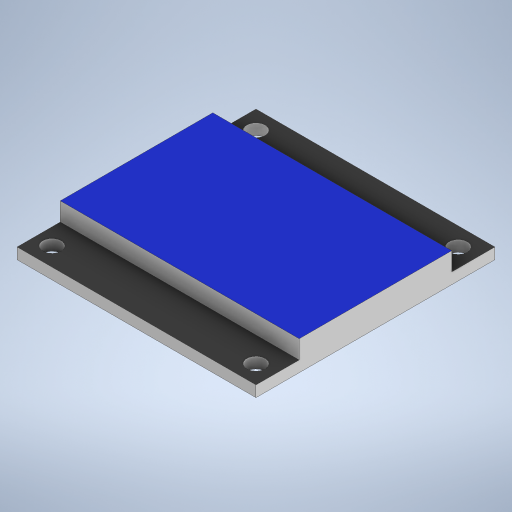
# Autodesk Inventor part: ssd1360
Saved by Autodesk Inventor 2023 (Build 270158000, 158)
## iProperties
Created: 2023-05-18
Part Number: ssd1360
Material: Generic
Document SubType Name: Modeling
Designer: mark
Density: 1 g/cm^3
Appearance: Default
Author: mark
Autodesk Inventor part; units mm, degrees
ref_plane "YZ Plane" through (0, 0, 0) normal (1, 0, 0) x (0, 1, 0)
ref_plane "XZ Plane" through (0, 0, 0) normal (0, 1, 0) x (-1, 0, 0)
ref_plane "XY Plane" through (0, 0, 0) normal (0, 0, 1) x (1, 0, 0)
sketch "Sketch1" plane through (0, 0, 0) normal (0, 1, 0) x (-1, 0, 0)
  line L0 (63.6448, -68.929) -> (37.6448, -68.929)
  line L1 (37.6448, -68.929) -> (37.6448, -42.929)
  line L2 (37.6448, -42.929) -> (63.6448, -42.929)
  line L3 (63.6448, -42.929) -> (63.6448, -68.929)
  point P0 (0, 0)
  dimension "d0" = 26
  dimension "d1" = 26
  constraints: 8 end point, 2 parallel, 1 horizontal, 1 perpendicular
  measures "d0" distance of L1.end L2.end
  measures "d1" distance of L0.end L1.end
extrude "Extrusion1" add sketch "Sketch1" along normal blind 1.2
sketch "Sketch2" plane through (0, 1.2, 0) normal (0, 1, 0) x (1, 0, 0)
  line L0 (-63.6448, 68.929) -> (-63.6448, 42.929) projected
  line L1 (-37.6448, 42.929) -> (-37.6448, 68.929) projected
  line L2 (-63.6448, 64.229) -> (-37.6448, 64.229)
  line L3 (-37.6448, 64.229) -> (-37.6448, 47.629)
  line L4 (-37.6448, 47.629) -> (-63.6448, 47.629)
  line L5 (-63.6448, 47.629) -> (-63.6448, 64.229)
  line L6 (-37.6448, 68.929) -> (-63.6448, 68.929) projected
  point P0 (0, 0)
  point P1 (-63.6448, 47.629)
  dimension "d4" = 4.7
  dimension "d5" = 16.6
  constraints: 8 end point, 2 parallel, 2 point on line, 1 horizontal, 1 perpendicular
  measures "d4" distance between parallel lines of L2 L6
  measures "d5" distance between parallel lines of L2 L4
extrude "Extrusion2" add sketch "Sketch2" along normal blind 2 contours L2 L1 L4 L0
sketch "Sketch3" plane through (0, 1.2, 0) normal (0, 1, 0) x (1, 0, 0)
  circle A0 centre (-61.6448, 66.929) radius 1
  circle A1 centre (-39.6448, 66.929) radius 1
  circle A2 centre (-39.6448, 44.929) radius 1
  circle A3 centre (-61.8448, 44.929) radius 1
  line L0 (-63.6448, 68.929) -> (-63.6448, 64.229) projected
  line L1 (-37.6448, 68.929) -> (-63.6448, 68.929) projected
  line L2 (-37.6448, 64.229) -> (-37.6448, 68.929) projected
  line L3 (-37.6448, 42.929) -> (-37.6448, 47.629) projected
  line L4 (-63.6448, 42.929) -> (-37.6448, 42.929) projected
  line L5 (-63.6448, 47.629) -> (-63.6448, 42.929) projected
  point P0 (0, 0)
  point P1 (-63.6448, 45.279)
  dimension "d8" = 2
  dimension "d9" = 2
  dimension "d10" = 2
  dimension "d11" = 2
  dimension "d12" = 2
  dimension "d13" = 2
  dimension "d14" = 2
  dimension "d15" = 2
  dimension "d16" = 2
  dimension "d17" = 2
  dimension "d18" = 2
  dimension "d19" = 1.8
  constraints: 4 centre point, 1 midpoint
  measures "d8" diameter of A0
  measures "d9" diameter of A1
  measures "d10" diameter of A2
  measures "d11" diameter of A3
  measures "d12" distance from line of L0 A0.centre
  measures "d13" distance from line of L1 A0.centre
  measures "d14" distance from line of L1 A1.centre
  measures "d15" distance from line of L2 A1.centre
  measures "d16" distance from line of L3 A2.centre
  measures "d17" distance from line of L4 A2.centre
  measures "d18" distance from line of L4 A3.centre
  measures "d19" horizontal distance of point (-63.645, 45.279) A3.centre
extrude "Extrusion3" cut sketch "Sketch3" against normal through all
sketch "Sketch4" plane through (0, 0, 0) normal (0, -1, 0) x (1, 0, 0)
  line L0 (-45.8948, -68.929) -> (-55.8948, -68.929)
  line L1 (-55.8948, -68.929) -> (-55.8948, -66.429)
  line L2 (-55.8948, -66.429) -> (-45.8948, -66.429)
  line L3 (-45.8948, -66.429) -> (-45.8948, -68.929)
  line L4 (-37.6448, -68.929) -> (-63.6448, -68.929) projected
  line L5 (-37.6448, -42.929) -> (-37.6448, -68.929) projected
  point P0 (0, 0)
  dimension "d22" = 10
  dimension "d23" = 2.5
  dimension "d24" = 0
  dimension "d25" = 8.25
  constraints: 8 end point, 2 parallel, 1 horizontal, 1 perpendicular
  measures "d22" distance of L1.end L2.end
  measures "d23" distance of L0.end L1.end
  measures "d24" distance between parallel lines of L4 L0
  measures "d25" distance between parallel lines of L5 L3
extrude "Extrusion4" add sketch "Sketch4" along normal blind 2.5
equation "\"d14\" = d13"
equation "\"d15\" = d14"
equation "\"d16\" = d14"
equation "\"d17\" = d15"
equation "\"d18\" = d12"
body "Solid1"
